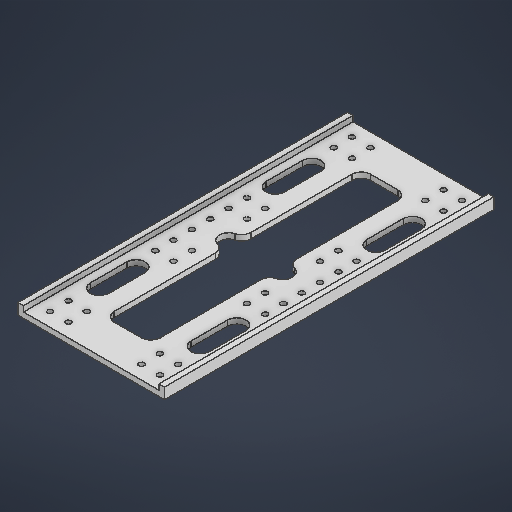
# Autodesk Inventor part: middle_base
Saved by Autodesk Inventor 2026.1 (Build 301233000, 233)
## iProperties
Created: 2026-03-10
Part Number: middle_base
Material: Generic
Document SubType Name: Modeling
Designer: emanuel
Density: 1 g/cm^3
Appearance: Default
Author: emanuel
Autodesk Inventor part; units mm, degrees
ref_plane "YZ Plane" through (0, 0, 0) normal (1, 0, 0) x (0, 1, 0)
ref_plane "XZ Plane" through (0, 0, 0) normal (0, 1, 0) x (-1, 0, 0)
ref_plane "XY Plane" through (0, 0, 0) normal (0, 0, 1) x (1, 0, 0)
sketch "Sketch1" plane through (0, 0, 0) normal (0, 1, 0) x (-1, 0, 0)
  line L0 (0, 0) -> (80, 0)
  line L1 (80, 0) -> (80, -180)
  line L2 (80, -180) -> (0, -180)
  line L3 (0, -180) -> (0, 0)
  line L4 (70, -65) -> (10, -65)
  line L5 (10, -65) -> (10, -115)
  line L6 (10, -115) -> (70, -115)
  line L7 (70, -115) -> (70, -65)
  line L8 (70, -65) -> (10, -115) construction
  line L9 (10, -65) -> (70, -115) construction
  line L10 (70, -75) -> (10, -75)
  line L11 (10, -75) -> (10, -105)
  line L12 (10, -105) -> (70, -105)
  line L13 (70, -105) -> (70, -75)
  line L14 (70, -75) -> (10, -105) construction
  line L15 (10, -75) -> (70, -105) construction
  line L16 (10, -85) -> (70, -85)
  line L17 (70, -85) -> (70, -95)
  line L18 (70, -95) -> (10, -95)
  line L19 (10, -95) -> (10, -85)
  line L20 (10, -85) -> (70, -95) construction
  line L21 (70, -85) -> (10, -95) construction
  circle A0 centre (70, -65) radius 1.5
  circle A1 centre (70, -75) radius 1.5
  circle A2 centre (70, -85) radius 1.5
  circle A3 centre (70, -95) radius 1.5
  circle A4 centre (70, -105) radius 1.5
  circle A5 centre (70, -115) radius 1.5
  circle A6 centre (10, -65) radius 1.5
  circle A7 centre (10, -75) radius 1.5
  circle A8 centre (10, -85) radius 1.5
  circle A9 centre (10, -95) radius 1.5
  circle A10 centre (10, -105) radius 1.5
  circle A11 centre (10, -115) radius 1.5
  line L22 (27.5, -20) -> (52.5, -20)
  line L23 (52.5, -20) -> (52.5, -160)
  line L24 (52.5, -160) -> (27.5, -160)
  line L25 (27.5, -160) -> (27.5, -20)
  line L26 (27.5, -20) -> (52.5, -160) construction
  line L27 (52.5, -20) -> (27.5, -160) construction
  line L28 (20, -65) -> (60, -65)
  line L29 (60, -65) -> (60, -115)
  line L30 (60, -115) -> (20, -115)
  line L31 (20, -115) -> (20, -65)
  line L32 (20, -65) -> (60, -115) construction
  line L33 (60, -65) -> (20, -115) construction
  circle A12 centre (60, -65) radius 1.5
  circle A13 centre (60, -115) radius 1.5
  circle A14 centre (20, -65) radius 1.5
  circle A15 centre (20, -115) radius 1.5
  circle A16 centre (60, -75) radius 1.5
  circle A17 centre (20, -75) radius 1.5
  circle A18 centre (60, -105) radius 1.5
  circle A19 centre (20, -105) radius 1.5
  point P0 (40, -90)
  point P1 (40, -90)
  point P2 (40, -90)
  point P3 (60, -85)
  point P4 (60, -95)
  point P5 (52.5, -95)
  point P6 (27.5, -95)
  point P7 (20, -95)
  point P8 (20, -85)
  point P9 (27.5, -85)
  point P10 (52.5, -85)
  dimension "d0" = 80
  dimension "d1" = 180
  dimension "d4" = 60
  dimension "d5" = 50
  dimension "d6" = 60
  dimension "d7" = 30
  dimension "d8" = 60
  dimension "d9" = 10
  dimension "d10" = 3
  dimension "d11" = 3
  dimension "d12" = 3
  dimension "d13" = 3
  dimension "d14" = 3
  dimension "d15" = 3
  dimension "d16" = 3
  dimension "d17" = 3
  dimension "d18" = 3
  dimension "d19" = 3
  dimension "d20" = 3
  dimension "d21" = 3
  dimension "d22" = 25
  dimension "d23" = 140
  dimension "d24" = 40
  dimension "d25" = 3
  dimension "d26" = 3
  dimension "d27" = 3
  dimension "d28" = 3
  dimension "d29" = 3
  dimension "d30" = 3
  dimension "d31" = 3
  dimension "d32" = 3
  constraints: 68 end point, 20 centre point, 12 midpoint, 12 parallel, 9 point on line, 6 horizontal, 6 perpendicular, 2 coincident
  measures "d0" distance of L1.end L2.end
  measures "d1" distance of L0.end L1.end
  measures "d4" distance of L6.end L5.end
  measures "d5" distance of L5.end L4.end
  measures "d6" distance of L12.end L11.end
  measures "d7" distance of L11.end L10.end
  measures "d8" distance of L17.end L18.end
  measures "d9" distance of L16.end L17.end
  measures "d10" diameter of A0
  measures "d11" diameter of A1
  measures "d12" diameter of A2
  measures "d13" diameter of A3
  measures "d14" diameter of A4
  measures "d15" diameter of A5
  measures "d16" diameter of A6
  measures "d17" diameter of A7
  measures "d18" diameter of A8
  measures "d19" diameter of A9
  measures "d20" diameter of A10
  measures "d21" diameter of A11
  measures "d22" distance of L23.end L24.end
  measures "d23" distance of L22.end L23.end
  measures "d24" distance of L29.end L30.end
  measures "d25" diameter of A12
  measures "d26" diameter of A13
  measures "d27" diameter of A14
  measures "d28" diameter of A15
  measures "d29" diameter of A16
  measures "d30" diameter of A17
  measures "d31" diameter of A18
  measures "d32" diameter of A19
extrude "Extrusion1" add sketch "Sketch1" along normal blind 3 contours L0 L1 L2 L3 | L4 A0 L7 A1 L10 A16 L29 A12 | A12 L29 A16 L10 L23 L4 | L25 L10 A17 L31 A14 L4 | L10 A16 L29 L16 L23 | L10 A1 L7 A2 L16 L29 A16 | L25 L16 L31 A17 L10 | A14 L31 A17 L10 A7 L5 A6 L4 | L16 A2 L7 A3 L18 L29 | L18 L29 A18 L12 L23 | L31 L16 A8 L5 A7 L10 A17 | L31 L18 A9 L5 A8 L16 | L25 L12 A19 L31 L18 | L18 A3 L7 A4 L12 A18 L29 | L12 A18 L29 A13 L6 L23 | L31 A19 L12 A10 L5 A9 L18 | L25 L6 A15 L31 A19 L12 | L12 A4 L7 A5 L6 A13 L29 A18 | A19 L31 A15 L6 A11 L5 A10 L12
fillet "Fillet1" radius 5 12 edges at (-52.5, 1.5, -160) (-27.5, 1.5, -160) (-60, 1.5, -95) (-52.5, 1.5, -95) (-60, 1.5, -85) (-52.5, 1.5, -85) (-52.5, 1.5, -20) (-27.5, 1.5, -20) (-27.5, 1.5, -85) (-20, 1.5, -85) (-20, 1.5, -95) (-27.5, 1.5, -95)
sketch "Sketch2" plane through (0, 3, 0) normal (0, 1, 0) x (1, 0, 0)
  line L0 (-80, 180) -> (-80, 0) projected
  line L1 (0, 0) -> (0, 180) projected
  line L2 (-80, 0) -> (0, 0)
  line L3 (0, 0) -> (0, 7.5)
  line L4 (0, 7.5) -> (-80, 7.5)
  line L5 (-80, 7.5) -> (-80, 0)
  line L6 (0, 7.5) -> (-80, 7.5)
  line L7 (-80, 7.5) -> (-80, 17.5)
  line L8 (-80, 17.5) -> (0, 17.5)
  line L9 (0, 17.5) -> (0, 7.5)
  line L10 (0, 180) -> (-80, 180) projected
  line L11 (-80, 180) -> (0, 180)
  line L12 (0, 180) -> (0, 172.5)
  line L13 (0, 172.5) -> (-80, 172.5)
  line L14 (-80, 172.5) -> (-80, 180)
  line L15 (0, 172.5) -> (-80, 172.5)
  line L16 (-80, 172.5) -> (-80, 162.5)
  line L17 (-80, 162.5) -> (0, 162.5)
  line L18 (0, 162.5) -> (0, 172.5)
  line L19 (-80, 0) -> (-70, 0)
  line L20 (-70, 0) -> (-70, 180)
  line L21 (-70, 180) -> (-80, 180)
  line L22 (-80, 180) -> (-80, 0)
  line L23 (0, 0) -> (-10, 0)
  line L24 (-10, 0) -> (-10, 180)
  line L25 (-10, 180) -> (0, 180)
  line L26 (0, 180) -> (0, 0)
  line L27 (-70, 0) -> (-60, 0)
  line L28 (-60, 0) -> (-60, 180)
  line L29 (-60, 180) -> (-70, 180)
  line L30 (-70, 180) -> (-70, 0)
  line L31 (-10, 0) -> (-20, 0)
  line L32 (-20, 0) -> (-20, 180)
  line L33 (-20, 180) -> (-10, 180)
  line L34 (-10, 180) -> (-10, 0)
  circle A0 centre (-70, 7.5) radius 1.5
  circle A1 centre (-70, 17.5) radius 1.5
  circle A2 centre (-60, 7.5) radius 1.5
  circle A3 centre (-60, 17.5) radius 1.5
  line L35 (0, 0) -> (-10, 0)
  line L36 (-10, 0) -> (-10, 7.5)
  line L37 (-10, 7.5) -> (0, 7.5)
  line L38 (0, 7.5) -> (0, 0)
  line L39 (0, 180) -> (-10, 180)
  line L40 (-10, 180) -> (-10, 162.5)
  line L41 (-10, 162.5) -> (0, 162.5)
  line L42 (0, 162.5) -> (0, 180)
  line L43 (-80, 180) -> (-70, 180)
  line L44 (-70, 180) -> (-70, 162.5)
  line L45 (-70, 162.5) -> (-80, 162.5)
  line L46 (-80, 162.5) -> (-80, 180)
  circle A4 centre (-70, 162.5) radius 1.5
  circle A5 centre (-70, 172.5) radius 1.5
  circle A6 centre (-60, 162.5) radius 1.5
  circle A7 centre (-60, 172.5) radius 1.5
  circle A8 centre (-20, 7.5) radius 1.5
  circle A9 centre (-20, 17.5) radius 1.5
  circle A10 centre (-10, 7.5) radius 1.5
  circle A11 centre (-10, 17.5) radius 1.5
  circle A12 centre (-20, 162.5) radius 1.5
  circle A13 centre (-20, 172.5) radius 1.5
  circle A14 centre (-10, 162.5) radius 1.5
  circle A15 centre (-10, 172.5) radius 1.5
  dimension "d34" = 7.5
  dimension "d35" = 10
  dimension "d36" = 7.5
  dimension "d37" = 10
  dimension "d38" = 10
  dimension "d39" = 10
  dimension "d40" = 10
  dimension "d41" = 10
  dimension "d42" = 3
  dimension "d43" = 3
  dimension "d44" = 3
  dimension "d45" = 3
  dimension "d46" = 3
  dimension "d47" = 3
  dimension "d48" = 3
  dimension "d49" = 3
  dimension "d50" = 3
  dimension "d51" = 3
  dimension "d52" = 3
  dimension "d53" = 3
  dimension "d54" = 3
  dimension "d55" = 3
  dimension "d56" = 3
  dimension "d57" = 3
  constraints: 88 end point, 22 parallel, 22 point on line, 16 centre point, 11 horizontal, 11 perpendicular
  measures "d34" distance of L3.end L2.end
  measures "d35" distance of L6.end L7.end
  measures "d36" distance of L11.end L12.end
  measures "d37" distance of L16.end L15.end
  measures "d38" distance of L21.end L20.end
  measures "d39" distance of L24.end L25.end
  measures "d40" distance of L29.end L28.end
  measures "d41" distance of L32.end L33.end
  measures "d42" diameter of A0
  measures "d43" diameter of A1
  measures "d44" diameter of A2
  measures "d45" diameter of A3
  measures "d46" diameter of A4
  measures "d47" diameter of A5
  measures "d48" diameter of A6
  measures "d49" diameter of A7
  measures "d50" diameter of A8
  measures "d51" diameter of A9
  measures "d52" diameter of A10
  measures "d53" diameter of A11
  measures "d54" diameter of A12
  measures "d55" diameter of A13
  measures "d56" diameter of A14
  measures "d57" diameter of A15
extrude "Extrusion2" cut sketch "Sketch2" against normal blind 3 contours A5 L20 L13 | L13 L20 A5 | A5 L13 L20 | A4 L20 L17 | L17 L20 A4 | L13 A5 L20 | A7 L13 L28 | L28 L13 A7 | A1 L20 L8 | L8 L20 A1 | L20 A4 L17 | L17 A4 L20 | A13 L13 L32 | L32 L13 A13 | L28 A7 L13 | L13 A7 L28 | A0 L20 L4 | L4 L20 A0 | L20 A1 L8 | L8 A1 L20 | A15 L13 L24 | L24 L13 A15 | L32 A13 L13 | L13 A13 L32 | L20 A0 L4 | L4 A0 L20 | A6 L28 L17 | L17 L28 A6 | L24 A15 L13 | L13 A15 L24 | A6 L17 L28 | A3 L28 L8 | L8 L28 A3 | L17 A6 L28 | A12 L17 L32 | L32 L17 A12 | A2 L4 L28 | L28 L4 A2 | A2 L28 L4 | L28 A3 L8 | L8 A3 L28 | A14 L24 L17 | L17 L24 A14 | L24 L17 A14 | L32 A12 L17 | L17 A12 L32 | A8 L4 L32 | L32 L4 A8 | L28 A2 L4 | A11 L24 L8 | L8 L24 A11 | L24 A14 L17 | A10 L4 L24 | L24 L4 A10 | L32 A8 L4 | L4 A8 L32 | A9 L32 L8 | L8 L32 A9 | L4 L24 A10 | L24 A11 L8 | L8 A11 L24 | A9 L8 L32 | L4 A10 L24 | L8 A9 L32
sketch "Sketch3" plane through (0, 3, 0) normal (0, 1, 0) x (1, 0, 0)
  line L0 (0, 180) -> (-80, 180) projected
  line L1 (0, 0) -> (-3, 0)
  line L2 (-3, 0) -> (-3, 180)
  line L3 (-3, 180) -> (0, 180)
  line L4 (0, 180) -> (0, 0)
  line L5 (-80, 180) -> (-80, 0) projected
  line L6 (-80, 180) -> (-77, 180)
  line L7 (-77, 180) -> (-77, 0)
  line L8 (-77, 0) -> (-80, 0)
  line L9 (-80, 0) -> (-80, 180)
  dimension "d60" = 3
  dimension "d61" = 3
  constraints: 16 end point, 4 parallel, 2 horizontal, 2 perpendicular, 2 point on line
  measures "d60" distance of L2.end L3.end
  measures "d61" distance of L7.end L8.end
extrude "Extrusion3" add sketch "Sketch3" along normal blind 3
sketch "Sketch4" plane through (0, 3, 0) normal (0, 1, 0) x (1, 0, 0)
  arc A0 (-52.5, 25) -> (-47.5, 20) centre (-47.5, 25) ccw projected
  line L0 (-47.5, 25) -> (-67.5, 25)
  line L1 (-67.5, 25) -> (-67.5, 42)
  line L2 (-67.5, 42) -> (-47.5, 42)
  line L3 (-47.5, 42) -> (-47.5, 25)
  arc A1 (-32.5, 20) -> (-27.5, 25) centre (-32.5, 25) ccw projected
  line L4 (-32.5, 25) -> (-12.5, 25)
  line L5 (-12.5, 25) -> (-12.5, 42)
  line L6 (-12.5, 42) -> (-32.5, 42)
  line L7 (-32.5, 42) -> (-32.5, 25)
  arc A2 (-47.5, 160) -> (-52.5, 155) centre (-47.5, 155) ccw projected
  line L8 (-47.5, 155) -> (-67.5, 155)
  line L9 (-67.5, 155) -> (-67.5, 138)
  line L10 (-67.5, 138) -> (-47.5, 138)
  line L11 (-47.5, 138) -> (-47.5, 155)
  arc A3 (-27.5, 155) -> (-32.5, 160) centre (-32.5, 155) ccw projected
  line L12 (-32.5, 155) -> (-12.5, 155)
  line L13 (-12.5, 155) -> (-12.5, 138)
  line L14 (-12.5, 138) -> (-32.5, 138)
  line L15 (-32.5, 138) -> (-32.5, 155)
  line L16 (-72.5, 123) -> (-62.5, 123)
  line L17 (-62.5, 123) -> (-62.5, 153)
  line L18 (-62.5, 153) -> (-72.5, 153)
  line L19 (-72.5, 153) -> (-72.5, 123)
  line L20 (-72.5, 123) -> (-62.5, 153) construction
  line L21 (-62.5, 123) -> (-72.5, 153) construction
  line L22 (-7.5, 123) -> (-17.5, 123)
  line L23 (-17.5, 123) -> (-17.5, 153)
  line L24 (-17.5, 153) -> (-7.5, 153)
  line L25 (-7.5, 153) -> (-7.5, 123)
  line L26 (-7.5, 123) -> (-17.5, 153) construction
  line L27 (-17.5, 123) -> (-7.5, 153) construction
  line L28 (-72.5, 57) -> (-62.5, 57)
  line L29 (-62.5, 57) -> (-62.5, 27)
  line L30 (-62.5, 27) -> (-72.5, 27)
  line L31 (-72.5, 27) -> (-72.5, 57)
  line L32 (-72.5, 57) -> (-62.5, 27) construction
  line L33 (-62.5, 57) -> (-72.5, 27) construction
  line L34 (-7.5, 57) -> (-17.5, 57)
  line L35 (-17.5, 57) -> (-17.5, 27)
  line L36 (-17.5, 27) -> (-7.5, 27)
  line L37 (-7.5, 27) -> (-7.5, 57)
  line L38 (-7.5, 57) -> (-17.5, 27) construction
  line L39 (-17.5, 57) -> (-7.5, 27) construction
  point P0 (0, 0)
  dimension "d64" = 20
  dimension "d65" = 17
  dimension "d66" = 20
  dimension "d67" = 17
  dimension "d68" = 20
  dimension "d69" = 17
  dimension "d70" = 20
  dimension "d71" = 17
  dimension "d72" = 10
  dimension "d73" = 30
  dimension "d74" = 10
  dimension "d75" = 30
  dimension "d76" = 10
  dimension "d77" = 30
  dimension "d78" = 10
  dimension "d79" = 30
  constraints: 80 end point, 16 parallel, 8 horizontal, 8 midpoint, 8 perpendicular
  measures "d64" distance of L1.end L2.end
  measures "d65" distance of L0.end L1.end
  measures "d66" distance of L6.end L5.end
  measures "d67" distance of L5.end L4.end
  measures "d68" distance of L10.end L9.end
  measures "d69" distance of L9.end L8.end
  measures "d70" distance of L13.end L14.end
  measures "d71" distance of L12.end L13.end
  measures "d72" distance of L18.end L17.end
  measures "d73" distance of L17.end L16.end
  measures "d74" distance of L23.end L24.end
  measures "d75" distance of L22.end L23.end
  measures "d76" distance of L29.end L30.end
  measures "d77" distance of L28.end L29.end
  measures "d78" distance of L36.end L35.end
  measures "d79" distance of L35.end L34.end
extrude "Extrusion4" cut sketch "Sketch4" against normal blind 3 contours L29 L30 L1 L2 | L2 L1 L30 L31 L28 L29 | L35 L34 L37 L36 L5 L6 | L6 L5 L36 L35 | L17 L16 L19 L18 L9 L10 | L10 L9 L18 L17 | L23 L24 L13 L14 | L14 L13 L24 L25 L22 L23
fillet "Fillet2" radius 5 16 edges at (-17.5, 1.5, -123) (-7.5, 1.5, -123) (-17.5, 1.5, -153) (-7.5, 1.5, -153) (-17.5, 1.5, -57) (-7.5, 1.5, -57) (-17.5, 1.5, -27) (-7.5, 1.5, -27) (-62.5, 1.5, -27) (-72.5, 1.5, -27) (-72.5, 1.5, -57) (-62.5, 1.5, -57) (-72.5, 1.5, -123) (-62.5, 1.5, -123) (-72.5, 1.5, -153) (-62.5, 1.5, -153)
body "Solid1"
